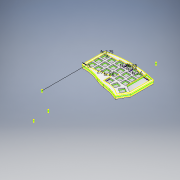
# Autodesk Inventor part: stacked curvy
Saved by Autodesk Inventor 2021 (Build 250183000, 183)
## iProperties
Created: 2021-11-19
Part Number: stacked curvy
Material: Polystyrene
Document SubType Name: Modeling
Designer: Mark
Density: 1.021 g/cm^3
Appearance: Smooth - White
Author: Mark
Autodesk Inventor part; units mm, degrees
ref_plane "YZ Plane" through (0, 0, 0) normal (1, 0, 0) x (0, 1, 0)
ref_plane "XZ Plane" through (0, 0, 0) normal (0, 1, 0) x (-1, 0, 0)
ref_plane "XY Plane" through (0, 0, 0) normal (0, 0, 1) x (1, 0, 0)
sketch "screw" plane through (0, 0, 0) normal (0, 0, 1) x (1, 0, 0)
  circle A0 centre (98.5317, 48.7492) radius 1.375 construction
  line L0 (96.7131, 45.5992) -> (94.8944, 48.7492) construction
  line L1 (94.8944, 48.7492) -> (96.7131, 51.8992) construction
  line L2 (96.7131, 51.8992) -> (100.3504, 51.8992) construction
  line L3 (100.3504, 51.8992) -> (102.169, 48.7492) construction
  line L4 (102.169, 48.7492) -> (100.3504, 45.5992) construction
  line L5 (100.3504, 45.5992) -> (96.7131, 45.5992) construction
  circle A1 centre (98.5317, 48.7492) radius 2.72 construction
  point P0 (98.5317, 48.7492)
  dimension "d32" = 2.75
  dimension "d34" = 6.3
  dimension "d35" = 5.44
  measures "d32" diameter of A0
  measures "d34" distance between parallel lines of L5 L2
  measures "d35" diameter of A1
sketch "Sketch1" plane through (0, 0, 0) normal (0, 1, 0) x (-1, 0, 0)
  line L0 (-42.2104, 23.6727) -> (-54.3348, 30.6727)
  line L1 (-54.3348, 30.6727) -> (-47.3348, 42.7971)
  line L2 (-47.3348, 42.7971) -> (-35.2104, 35.7971)
  line L3 (-35.2104, 35.7971) -> (-42.2104, 23.6727)
  line L4 (-23.0354, 2.5115) -> (-37.0354, 2.5115)
  line L5 (-37.0354, 2.5115) -> (-37.0354, 16.5115)
  line L6 (-37.0354, 16.5115) -> (-23.0354, 16.5115)
  line L7 (-23.0354, 16.5115) -> (-23.0354, 2.5115)
  line L8 (-20.5336, -37.8635) -> (-39.0203, -37.8635)
  line L9 (-23.0354, -21.4885) -> (-23.0354, -35.4885)
  line L10 (-23.0354, -35.4885) -> (-37.0354, -35.4885)
  line L11 (-37.0354, -35.4885) -> (-37.0354, -21.4885)
  line L12 (-37.0354, -21.4885) -> (-23.0354, -21.4885)
  line L13 (-37.0354, -16.4885) -> (-37.0354, -2.4885)
  line L14 (-37.0354, -2.4885) -> (-23.0354, -2.4885)
  line L15 (-23.0354, -2.4885) -> (-23.0354, -16.4885)
  line L16 (-23.0354, -16.4885) -> (-37.0354, -16.4885)
  line L17 (-59.4168, -33.9899) -> (-39.0203, -33.9899)
  line L18 (-27.4644, 38.068) -> (-13.9414, 34.4445)
  line L19 (-13.9414, 34.4445) -> (-17.5649, 20.9215)
  line L20 (-17.5649, 20.9215) -> (-31.0878, 24.545)
  line L21 (-31.0878, 24.545) -> (-27.4644, 38.068)
  line L22 (-11.1658, 36.1596) -> (-29.1483, 40.978)
  line L23 (52.9698, -19.1242) -> (52.9698, -33.1242)
  line L24 (52.9698, -33.1242) -> (38.9698, -33.1242)
  line L25 (38.9698, -33.1242) -> (38.9698, -19.1242)
  line L26 (38.9698, -19.1242) -> (52.9698, -19.1242)
  line L27 (19.9695, -18.8691) -> (19.9695, -4.8691)
  line L28 (19.9695, -4.8691) -> (33.9695, -4.8691)
  line L29 (33.9695, -4.8691) -> (33.9695, -18.8691)
  line L30 (33.9695, -18.8691) -> (19.9695, -18.8691)
  line L31 (-18.0336, 14.1267) -> (-4.0336, 14.1267)
  line L32 (-4.0336, 14.1267) -> (-4.0336, 0.1267)
  line L33 (-4.0336, 0.1267) -> (-18.0336, 0.1267)
  line L34 (-18.0336, 0.1267) -> (-18.0336, 14.1267)
  line L35 (5.448, 33.7846) -> (5.448, 19.7846)
  line L36 (5.448, 19.7846) -> (-8.552, 19.7846)
  line L37 (-8.552, 19.7846) -> (-8.552, 33.7846)
  line L38 (-8.552, 33.7846) -> (5.448, 33.7846)
  line L39 (7.823, 14.1271) -> (7.823, 36.1596)
  line L40 (33.9695, 0.1309) -> (19.9695, 0.1309)
  line L41 (19.9695, 0.1309) -> (19.9695, 14.1309)
  line L42 (19.9695, 14.1309) -> (33.9695, 14.1309)
  line L43 (33.9695, 14.1309) -> (33.9695, 0.1309)
  line L44 (71.968, -14.1236) -> (57.968, -14.1236)
  line L45 (57.968, -14.1236) -> (57.968, -0.1236)
  line L46 (57.968, -0.1236) -> (71.968, -0.1236)
  line L47 (71.968, -0.1236) -> (71.968, -14.1236)
  line L48 (52.9698, 18.8757) -> (52.9698, 4.8757)
  line L49 (52.9698, 4.8757) -> (38.9698, 4.8757)
  line L50 (38.9698, 4.8757) -> (38.9698, 18.8757)
  line L51 (38.9698, 18.8757) -> (52.9698, 18.8757)
  line L52 (57.968, -19.1236) -> (71.968, -19.1236)
  line L53 (71.968, -19.1236) -> (71.968, -33.1236)
  line L54 (71.968, -33.1236) -> (57.968, -33.1236)
  line L55 (57.968, -33.1236) -> (57.968, -19.1236)
  line L56 (36.3698, 16.5059) -> (17.3695, 16.5059)
  line L57 (33.9695, -37.8691) -> (19.9695, -37.8691)
  line L58 (19.9695, -37.8691) -> (19.9695, -23.8691)
  line L59 (19.9695, -23.8691) -> (33.9695, -23.8691)
  line L60 (33.9695, -23.8691) -> (33.9695, -37.8691)
  line L61 (57.968, 18.8764) -> (71.968, 18.8764)
  line L62 (71.968, 18.8764) -> (71.968, 4.8764)
  line L63 (71.968, 4.8764) -> (57.968, 4.8764)
  line L64 (57.968, 4.8764) -> (57.968, 18.8764)
  line L65 (36.4695, -35.4992) -> (36.4695, -40.2441)
  line L66 (14.9676, -26.2479) -> (14.9676, -40.2479)
  line L67 (14.9676, -40.2479) -> (0.9676, -40.2479)
  line L68 (0.9676, -40.2479) -> (0.9676, -26.2479)
  line L69 (0.9676, -26.2479) -> (14.9676, -26.2479)
  line L70 (36.3695, -40.2441) -> (17.5676, -40.2441)
  line L71 (14.9676, -7.2479) -> (14.9676, -21.2479)
  line L72 (14.9676, -21.2479) -> (0.9676, -21.2479)
  line L73 (0.9676, -21.2479) -> (0.9676, -7.2479)
  line L74 (0.9676, -7.2479) -> (14.9676, -7.2479)
  line L75 (-39.0354, -0.6821) -> (-39.0354, -18.6821)
  line L76 (-20.6336, -40.2483) -> (-20.6336, -37.8635)
  line L77 (0.9676, 11.7521) -> (14.9676, 11.7521)
  line L78 (14.9676, 11.7521) -> (14.9676, -2.2479)
  line L79 (14.9676, -2.2479) -> (0.9676, -2.2479)
  line L80 (0.9676, -2.2479) -> (0.9676, 11.7521)
  line L81 (7.823, 36.1596) -> (-11.1658, 36.1596)
  line L82 (-4.0336, -4.8733) -> (-4.0336, -18.8733)
  line L83 (-4.0336, -18.8733) -> (-18.0336, -18.8733)
  line L84 (-18.0336, -18.8733) -> (-18.0336, -4.8733)
  line L85 (-18.0336, -4.8733) -> (-4.0336, -4.8733)
  line L86 (-1.6324, -42.6229) -> (-1.6324, -40.2483)
  line L87 (-4.0336, -23.8733) -> (-4.0336, -37.8733)
  line L88 (-4.0336, -37.8733) -> (-18.0336, -37.8733)
  line L89 (-18.0336, -37.8733) -> (-18.0336, -23.8733)
  line L90 (-18.0336, -23.8733) -> (-4.0336, -23.8733)
  line L91 (17.5676, -42.6229) -> (-1.5324, -42.6229)
  line L92 (-45.63, 50.4998) -> (-29.1483, 40.978)
  line L93 (-1.5324, -40.2483) -> (-20.5336, -40.2483)
  line L94 (52.9698, -0.1243) -> (52.9698, -14.1243)
  line L95 (52.9698, -14.1243) -> (38.9698, -14.1243)
  line L96 (38.9698, -14.1243) -> (38.9698, -0.1243)
  line L97 (38.9698, -0.1243) -> (52.9698, -0.1243)
  line L98 (-39.0201, 14.9026) -> (-39.0203, -33.9899)
  line L99 (-37.0354, -21.4885) -> (-23.0354, -21.4885)
  line L100 (-23.0354, -21.4885) -> (-23.0354, -35.4885)
  line L101 (-23.0354, -35.4885) -> (-37.0354, -35.4885)
  line L102 (-37.0354, -35.4885) -> (-37.0354, -21.4885)
  line L103 (-39.0203, -43.5464) -> (-39.0204, 14.9027)
  line L104 (17.3695, 14.1271) -> (7.723, 14.1271)
  line L105 (17.3695, 16.5059) -> (17.3695, 14.1271)
  line L106 (74.343, -35.4992) -> (36.4695, -35.4992)
  line L107 (17.5676, -40.2441) -> (17.5676, -42.6229)
  line L108 (36.3698, 21.2514) -> (36.3698, 16.5059)
  line L109 (-39.0201, 14.9026) -> (-59.3916, 26.6641)
  arc A0 (21.9963, 32.5167) -> (74.343, 21.2514) centre (74.343, 148.5046) ccw
  arc A1 (-59.4168, -33.9899) -> (74.343, -35.4992) centre (10.5172, 235.9081) ccw
  line L110 (36.3698, 21.2514) -> (74.343, 21.2514)
  line L111 (71.968, 21.2514) -> (74.343, 21.2514)
  line L112 (-45.63, 50.4998) -> (-59.4283, 26.6004)
  line L113 (-59.4283, 26.6004) -> (-59.4158, -39.1522)
  line L114 (74.343, -35.4992) -> (74.343, 21.2514)
  arc A2 (-45.63, 50.4998) -> (-3.1171, 39.2971) centre (13.8917, 190.1106) ccw
  arc A3 (21.9963, 32.5167) -> (-3.1171, 39.2971) centre (-23.6416, -86.6203) ccw
  arc A4 (-64.4161, -37.8323) -> (79.343, -39.4313) centre (10.5172, 235.9081) ccw
  line L115 (-64.4161, -37.8323) -> (-64.4286, 27.9397)
  line L116 (-64.4286, 27.9397) -> (-47.7113, 56.895)
  arc A5 (-47.7113, 56.895) -> (-2.4366, 44.2521) centre (13.8917, 190.1106) ccw
  arc A6 (23.9232, 37.1328) -> (-2.4366, 44.2521) centre (-23.6416, -86.6203) ccw
  arc A7 (23.9232, 37.1328) -> (79.343, 26.3537) centre (74.343, 148.5046) ccw
  line L117 (79.343, 26.3537) -> (79.343, -39.4313)
  arc A8 (-61.9164, -35.9178) -> (76.843, -37.4724) centre (10.5172, 235.9081) ccw construction
  line L118 (-61.9164, -35.9178) -> (-61.9285, 27.2701) construction
  line L119 (-61.9285, 27.2701) -> (-46.6792, 53.6826) construction
  arc A9 (-46.6792, 53.6826) -> (-2.7763, 41.7745) centre (13.8917, 190.1106) ccw construction
  arc A10 (22.9591, 34.825) -> (-2.7763, 41.7745) centre (-23.6416, -86.6203) ccw construction
  arc A11 (22.9591, 34.825) -> (76.843, 23.7765) centre (74.343, 148.5046) ccw construction
  line L120 (76.843, 23.7765) -> (76.843, -37.4724) construction
  circle A12 centre (69.4904, -39.1522) radius 1.375
  circle A13 centre (76.843, 23.7765) radius 1.375 construction
  line L121 (75.0243, 20.6265) -> (73.2057, 23.7765) construction
  line L122 (73.2057, 23.7765) -> (75.0243, 26.9265) construction
  line L123 (75.0243, 26.9265) -> (78.6616, 26.9265) construction
  line L124 (78.6616, 26.9265) -> (80.4803, 23.7765) construction
  line L125 (80.4803, 23.7765) -> (78.6616, 20.6265) construction
  line L126 (78.6616, 20.6265) -> (75.0243, 20.6265) construction
  circle A14 centre (76.843, 23.7765) radius 2.72 construction
  circle A15 centre (-46.6792, 53.6826) radius 1.375 construction
  line L127 (-48.4978, 50.5326) -> (-50.3165, 53.6826) construction
  line L128 (-50.3165, 53.6826) -> (-48.4978, 56.8326) construction
  line L129 (-48.4978, 56.8326) -> (-44.8605, 56.8326) construction
  line L130 (-44.8605, 56.8326) -> (-43.0419, 53.6826) construction
  line L131 (-43.0419, 53.6826) -> (-44.8605, 50.5326) construction
  line L132 (-44.8605, 50.5326) -> (-48.4978, 50.5326) construction
  circle A16 centre (-46.6792, 53.6826) radius 2.72 construction
  circle A17 centre (76.843, -37.4724) radius 1.375 construction
  line L133 (75.0243, -40.6224) -> (73.2057, -37.4724) construction
  line L134 (73.2057, -37.4724) -> (75.0243, -34.3224) construction
  line L135 (75.0243, -34.3224) -> (78.6616, -34.3224) construction
  line L136 (78.6616, -34.3224) -> (80.4803, -37.4724) construction
  line L137 (80.4803, -37.4724) -> (78.6616, -40.6224) construction
  line L138 (78.6616, -40.6224) -> (75.0243, -40.6224) construction
  circle A18 centre (76.843, -37.4724) radius 2.72 construction
  circle A19 centre (-61.9164, -35.9178) radius 1.375 construction
  line L139 (-63.7351, -39.0678) -> (-65.5538, -35.9178) construction
  line L140 (-65.5538, -35.9178) -> (-63.7351, -32.7678) construction
  line L141 (-63.7351, -32.7678) -> (-60.0978, -32.7678) construction
  line L142 (-60.0978, -32.7678) -> (-58.2791, -35.9178) construction
  line L143 (-58.2791, -35.9178) -> (-60.0978, -39.0678) construction
  line L144 (-60.0978, -39.0678) -> (-63.7351, -39.0678) construction
  circle A20 centre (-61.9164, -35.9178) radius 2.72 construction
  point P0 (0, 0)
  point P1 (-39.0203, -33.9899)
  point P2 (38.9698, -0.1243)
  point P3 (14.9676, -2.2479)
  point P4 (0.9676, -21.2479)
  point P5 (0.9676, -40.2479)
  point P6 (71.968, 4.8764)
  point P7 (52.9698, 4.8757)
  point P8 (57.968, -0.1236)
  point P9 (-8.552, 19.7846)
  point P10 (-4.0336, 0.1267)
  point P11 (19.9695, -4.8691)
  point P12 (-37.0354, -2.4885)
  point P13 (-49.2186, -33.9899)
  point P14 (-39.0203, -33.9899)
  dimension "d13" = 0
  dimension "d15" = 5
  dimension "d21" = 2.6
  dimension "d22" = 2.6
  dimension "d23" = 2.6
  dimension "d24" = 2.6
  dimension "d27" = 2.5
  dimension "d28" = 2.75
  dimension "d36" = 2.6
  constraints: 242 end point, 27 point on circle, 13 centre point, 10 vertical, 4 point on line, 2 horizontal, 1 midpoint, 17 other
  measures "d13" distance from line of L114 A0.centre
  measures "d15" radial gap between concentric circles of A1 A4
  measures "d21" distance between parallel lines of L86 L68
  measures "d22" distance between parallel lines of L76 L89
  measures "d23" distance between parallel lines of L108 L50
  measures "d24" distance between parallel lines of L105 L41
  measures "d27" radial gap between concentric circles of A4 A8
  measures "d28" diameter of A12
  measures "d36" distance between parallel lines of L107 L66
extrude "plate" add sketch "Sketch1" along normal blind 3.175 contours L113 A4 L115 L116 A5 A6 A7 L117 L103 A1 L114 A0 A3 A2 L112 | L98 L109 L112 L92 L22 L81 L39 L104 L105 L56 L108 L110 L114 A1 L103 | L110 L108 L56 L105 L104 L39 L81 L22 L92 A2 A3 A0 | A12
extrude "Extrusion5" add sketch "Sketch1" against normal blind 3.175 contours L113 A4 L115 L116 A5 A6 A7 L117 L103 A1 L114 A0 A3 A2 L112 | A1 L103 A4 L113 | A12
sketch "Sketch4" plane through (0, -3.175, 0) normal (0, -1, 0) x (1, 0, 0)
  arc A0 (-79.343, -39.4313) -> (64.4161, -37.8323) centre (-10.5172, 235.9081) ccw projected
  line L0 (64.4161, -37.8323) -> (64.4286, 27.9397) projected
  line L1 (64.4286, 27.9397) -> (47.7113, 56.895) projected
  arc A1 (2.4366, 44.2521) -> (47.7113, 56.895) centre (-13.8917, 190.1106) ccw projected
  arc A2 (2.4366, 44.2521) -> (-23.9232, 37.1328) centre (23.6416, -86.6203) ccw projected
  arc A3 (-79.343, 26.3537) -> (-23.9232, 37.1328) centre (-74.343, 148.5046) ccw projected
  line L2 (-79.343, 26.3537) -> (-79.343, -39.4313) projected
  line L3 (59.4283, 26.6004) -> (59.4168, -33.9899) projected
  arc A4 (-74.343, -35.4992) -> (59.4168, -33.9899) centre (-10.5172, 235.9081) ccw projected
  line L4 (-74.343, -35.4992) -> (-74.343, 21.2514) projected
  arc A5 (-74.343, 21.2514) -> (-21.9963, 32.5167) centre (-74.343, 148.5046) ccw projected
  arc A6 (3.1171, 39.2971) -> (-21.9963, 32.5167) centre (23.6416, -86.6203) ccw projected
  arc A7 (3.1171, 39.2971) -> (45.63, 50.4998) centre (-13.8917, 190.1106) ccw projected
  line L5 (45.63, 50.4998) -> (59.4283, 26.6004) projected
  point P0 (0, 0)
extrude "Extrusion6" add sketch "Sketch4" along normal blind 3.175 contours L2 A3 A2 A1 L1 L0 A0 | L3 A4 L4 A5 A6 A7 L5
sketch "Sketch5" plane through (0, 3.175, 0) normal (0, 1, 0) x (1, 0, 0)
  line L0 (-36.3695, 40.2441) -> (-17.5676, 40.2441) projected
  line L1 (-74.343, 35.4992) -> (-36.4695, 35.4992) projected
  line L2 (-36.4695, 35.4992) -> (-36.4695, 40.2441) projected
  line L3 (-17.5676, 40.2441) -> (-17.5676, 42.6229) projected
  line L4 (-17.5676, 42.6229) -> (1.5324, 42.6229) projected
  line L5 (1.6324, 42.6229) -> (1.6324, 40.2483) projected
  line L6 (1.5324, 40.2483) -> (20.5336, 40.2483) projected
  line L7 (20.6336, 40.2483) -> (20.6336, 37.8635) projected
  line L8 (20.5336, 37.8635) -> (39.0203, 37.8635) projected
  line L9 (39.0203, 43.5464) -> (39.0204, -14.9027) projected
  line L10 (59.4168, 33.9899) -> (39.0203, 33.9899) projected
  line L11 (59.4283, -26.6004) -> (59.4168, 33.9899) projected
  line L12 (45.63, -50.4998) -> (59.4283, -26.6004) projected
  line L13 (-74.343, 35.4992) -> (-74.343, -21.2514) projected
  arc A0 (64.4161, 37.8323) -> (-79.343, 39.4313) centre (-10.5172, -235.9081) ccw projected
  line L14 (64.4286, -27.9397) -> (64.4161, 37.8323) projected
  line L15 (47.7113, -56.895) -> (64.4286, -27.9397) projected
  arc A1 (47.7113, -56.895) -> (2.4366, -44.2521) centre (-13.8917, -190.1106) ccw projected
  arc A2 (-23.9232, -37.1328) -> (2.4366, -44.2521) centre (23.6416, 86.6203) ccw projected
  arc A3 (-23.9232, -37.1328) -> (-79.343, -26.3537) centre (-74.343, -148.5046) ccw projected
  line L16 (-79.343, 39.4313) -> (-79.343, -26.3537) projected
  line L17 (-36.3698, -21.2514) -> (-74.343, -21.2514) projected
  line L18 (-36.3698, -21.2514) -> (-36.3698, -16.5059) projected
  line L19 (-36.3698, -16.5059) -> (-17.3695, -16.5059) projected
  line L20 (-7.823, -14.1271) -> (-7.823, -36.1596) projected
  line L21 (-17.3695, -14.1271) -> (-7.723, -14.1271) projected
  line L22 (-17.3695, -16.5059) -> (-17.3695, -14.1271) projected
  line L23 (-7.823, -36.1596) -> (11.1658, -36.1596) projected
  line L24 (11.1658, -36.1596) -> (29.1483, -40.978) projected
  line L25 (45.63, -50.4998) -> (29.1483, -40.978) projected
  point P0 (0, 0)
  point P1 (39.0203, 37.8635)
  point P2 (39.0203, 33.9899)
  constraints: 6 other
extrude "Extrusion7" [suppressed]
equation "\"d32\" = screwhole"
equation "\"d34\" = nutsize"
equation "\"d35\" = screwhead"
equation "\"d15\" = wall"
equation "\"d21\" = d23"
equation "\"d22\" = d23"
equation "\"d24\" = d23"
equation "\"d27\" = 0.5 * wall"
equation "\"d28\" = screwhole"
equation "\"d36\" = d21"
equation "\"wall\" = 5"
equation "\"screwhole\" = 2.75"
equation "\"nutsize\" = 6.3"
equation "\"screwhead\" = 5.44"
body "Solid1"
